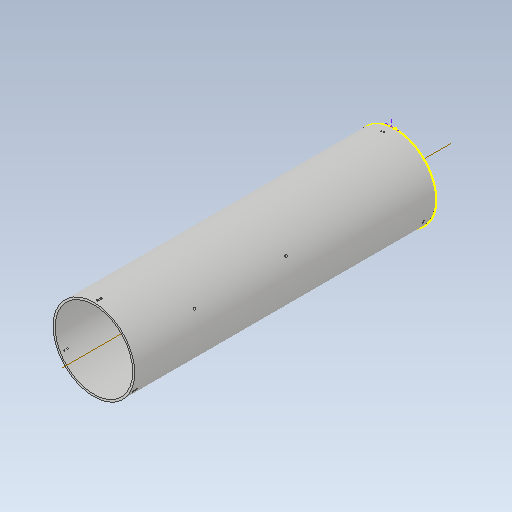
# Autodesk Inventor part: tuba2
Saved by Autodesk Inventor 2020 (Build 240168000, 168)
## iProperties
Created: 2019-05-25
Part Number: tuba2
Material: Ogólne
Document SubType Name: Modeling
Designer: Esterka
Density: 1 g/cm^3
Appearance: Domyślne
Author: Esterka
Autodesk Inventor part; units mm, degrees
sketch "Sketch1" plane through (0, 0, 0) normal (0, 0, 1) x (1, 0, 0)
  circle A0 centre (0, 0) radius 125
  circle A1 centre (0, 0) radius 118.7
  dimension "d0" = 250
  dimension "d1" = 237.4
  constraints: 2 centre point, 2 coincident
  measures "d0" diameter of A0
  measures "d1" diameter of A1
extrude "Extrusion1" add sketch "Sketch1" along normal blind 922
sketch "Sketch2" plane through (0, 0, 0) normal (0, 1, 0) x (-1, 0, 0)
  line L0 (-175, 0) -> (175, 0) projected
  point P0 (0, 0)
  point P1 (0, 6)
  dimension "d0" = 250
  dimension "d1" = 237.4
  dimension "d4" = 6
  measures "d4" distance from line of L0 point (0, 6)
ref_plane "Work Plane1" through (0, 0, 6) normal (0, 0, 1) x (1, 0, 0)
sketch "Sketch3" plane through (0, 0, 6) normal (0, 0, 1) x (1, 0, 0)
  circle A0 centre (0, 0) radius 125 projected
  point P0 (0, 125)
  point P1 (-108.2532, -62.5)
  point P2 (108.2532, -62.5)
  dimension "d7" = 360
  constraints: 1 vertical alignment, 5 other
ref_plane "Work Plane2" through (0, 125, 6) normal (0, 1, 0) x (-1, 0, 0)
sketch "Sketch4" plane through (0, 125, 6) normal (0, 1, 0) x (-1, 0, 0)
  line L0 (24, 20) -> (15.5, 20)
  line L1 (15.5, 20) -> (8.5, 20)
  line L2 (-125, -6) -> (125, -6) projected
  line L3 (0, -6) -> (0, 8.5799)
  dimension "d10" = 7
  dimension "d21" = 26
  dimension "d22" = 8.5
  constraints: 6 end point, 2 coincident, 1 horizontal, 1 point on line, 1 vertical
  measures "d10" distance of L0.end L1.end
  measures "d21" distance from line of L2 L1.end
  measures "d22" distance from line of point (8.5, 20) L3
hole "Hole1" at (-8.5, 125, 26) at (-15.5, 125, 26) direction (0, -1, 0) diameter 3.4 depth 8 tip angle 118 clearance for "Slotted Cheese Head Screw ISO 1207" size "M3" standard "ISO"
sketch "Sketch5" plane through (0, 125, 6) normal (0, 1, 0) x (-1, 0, 0)
  point P0 (0, -6)
ref_plane "Płaszczyzna konstrukcyjna3" through (0, 125, 0) normal (0, 1, 0) x (-1, 0, 0)
sketch "Szkic6" plane through (0, 125, 0) normal (0, 1, 0) x (-1, 0, 0)
  line L0 (125, 922) -> (-125, 922) projected
  point P0 (0, 0)
  point P1 (0, 910)
  point P2 (0, 900)
  dimension "d27" = 12
  dimension "d28" = 10
  measures "d27" distance from line of L0 point (0, 910)
  measures "d28" distance of point (0, 900) point (0, 910)
hole "Otwór2" at (0, 125, 910) at (0, 125, 900) direction (0, -1, 0) diameter 3.4 depth 8 tip angle 118 clearance for "Śruba ze łbem płaskim obrobiona" size "M3" standard "ANSI Profil metryczny M"
pattern_circular "Szyk kołowy3" count 3 over 360 about axis through (0, 0, -10) along (0, 0, 1) of "Otwór2"
chamfer "Faza1" distance 1.5 angle 45 12 edges at (-107.3932, -63.9665, 910.0006) (-109.0893, -61.0288, 909.8369) (-107.3932, -63.9665, 900.0006) (-109.0893, -61.0288, 899.8369) (109.0932, -61.022, 910.0006) (107.3972, -63.9597, 909.8369) (109.0932, -61.022, 900.0006) (107.3972, -63.9597, 899.8369) (-1.7, 124.9884, 910.0006) (1.6922, 124.9885, 909.8369) (-1.7, 124.9884, 900.0006) (1.6922, 124.9885, 899.8369)
ref_plane "Płaszczyzna konstrukcyjna4" through (108.2532, -62.5, 896.8) normal (0.866, -0.5, 0) x (0.5, 0.866, 0)
sketch "Szkic8" plane through (0, 0, 0) normal (0, 0, -1) x (-1, 0, 0)
  circle A0 centre (0, 0) radius 125 projected
  circle A1 centre (0, 0) radius 125 projected
  point P0 (0, -125)
  point P1 (11.2796, 124.49)
  constraints: 1 point on circle, 1 vertical alignment, 1 other
ref_plane "Płaszczyzna konstrukcyjna5" through (0, -125, 0) normal (0, -1, 0) x (1, 0, 0)
sketch "Szkic9" plane through (0, -125, 0) normal (0, -1, 0) x (1, 0, 0)
  line L0 (35.5, 24) -> (-35.5, 24)
  line L1 (-35.5, 24) -> (-35.5, 95)
  line L2 (-35.5, 95) -> (35.5, 95)
  line L3 (35.5, 95) -> (35.5, 24)
  line L4 (35.5, 24) -> (-35.5, 95) construction
  line L5 (-35.5, 24) -> (35.5, 95) construction
  line L6 (27.5, 32) -> (-27.5, 32)
  line L7 (-27.5, 32) -> (-27.5, 87)
  line L8 (-27.5, 87) -> (27.5, 87)
  line L9 (27.5, 87) -> (27.5, 32)
  line L10 (27.5, 32) -> (-27.5, 87) construction
  line L11 (-27.5, 32) -> (27.5, 87) construction
  circle A0 centre (0, 59.5) radius 27.5
  point P0 (0, 0)
  dimension "d51" = 59.5
  dimension "d52" = 71
  dimension "d53" = 71
  dimension "d54" = 55
  constraints: 24 end point, 5 coincident, 4 midpoint, 4 parallel, 2 horizontal, 2 perpendicular, 1 centre point, 1 point on line
  measures "d51" distance of point (0, 0) point (0, 59.5)
  measures "d52" distance of L1.end L2.end
  measures "d53" distance of L0.end L1.end
  measures "d54" distance of L7.end L8.end
hole "Otwór4" at (-35.5, -125, 24) at (-35.5, -125, 95) at (35.5, -125, 95) at (35.5, -125, 24) direction (0, 1, 0) diameter 6.756 depth 20 tip angle 118 clearance for "Śruba ze łbem płaskim obrobiona (82)" size "1/4" standard "ANSI Gwinty cal zunifikowane"
sketch "Szkic10" plane through (0, 0, 0) normal (0, 0, -1) x (-1, 0, 0)
  circle A0 centre (0, 0) radius 125 projected
  point P0 (-108.2532, 62.5)
  point P1 (-125, 0)
  dimension "d64" = 30
  constraints: 2 point on circle
ref_plane "Płaszczyzna konstrukcyjna6" through (108.2532, 62.5, 0) normal (0.866, 0.5, 0) x (-0.5, 0.866, 0)
sketch "Szkic11" plane through (108.2532, 62.5, 0) normal (0.866, 0.5, 0) x (-0.5, 0.866, 0)
  line L0 (0, 0) -> (0, 1115.0058)
  line L1 (125, 922) -> (-125, 922) projected
  point P0 (0, 722)
  point P1 (0, 442)
  dimension "d65" = 280
  dimension "d66" = 200
  constraints: 2 end point, 2 point on line, 1 vertical
  measures "d65" distance of point (0, 442) point (0, 722)
  measures "d66" distance from line of L1 point (0, 722)
hole "Otwór5" at (108.2532, 62.5, 442) at (108.2532, 62.5, 722) direction (-0.866, -0.5, 0) diameter 6.756 depth 20 tip angle 118 clearance for "Śruba ze łbem płaskim obrobiona (82)" size "1/4" standard "ANSI Gwinty cal zunifikowane"
extrude "Wyciągnięcie proste3" cut sketch "Szkic9" against normal blind 10 contours A0
ref_plane "Płaszczyzna konstrukcyjna8" through (-11.2796, 124.49, 0) normal (-0.0902, 0.9959, 0) x (-0.9959, -0.0902, 0)
sketch "Szkic13" plane through (-11.2796, 124.49, 0) normal (-0.0902, 0.9959, 0) x (-0.9959, -0.0902, 0)
  circle A0 centre (-2.7471, 26) radius 1.7
  circle A1 centre (4.2529, 26) radius 1.7
  point P0 (0, 0)
  dimension "d76" = 7
  dimension "d77" = 26
  dimension "d78" = 3.4
  dimension "d79" = 3.4
  constraints: 2 centre point
  measures "d76" distance of A0.centre A1.centre
  measures "d77" vertical distance of A0.centre point (0, 0)
  measures "d78" diameter of A0
  measures "d79" diameter of A1
extrude "Wyciągnięcie proste4" cut sketch "Szkic13" against normal blind 10
pattern_circular "Szyk kołowy4" count 3 over 360 about axis through (0, 0, -10) along (0, 0, 1) of "Wyciągnięcie proste4"
body "Solid1"
